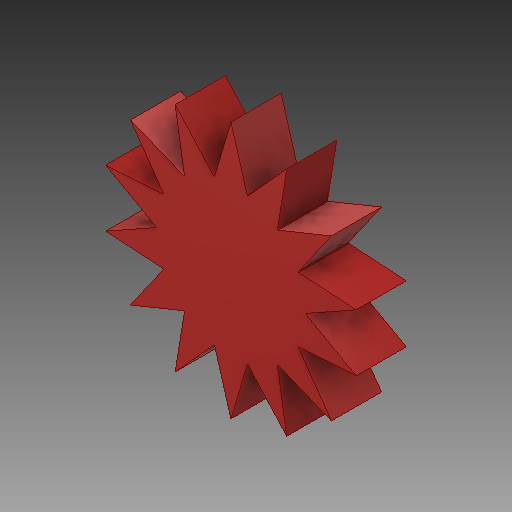
# Autodesk Inventor part: Small Gear Phone Case Mech
Saved by Autodesk Inventor 2018 (Build 220112000, 112)
## iProperties
Created: 2018-09-18
Part Number: Small Gear Phone Case Mech
Material: Generic
Document SubType Name: Modeling
Designer: User
Density: 1 g/cm^3
Appearance: Orange-Red
Author: User
Autodesk Inventor part; units mm, degrees
ref_plane "YZ Plane" through (0, 0, 0) normal (1, 0, 0) x (0, 1, 0)
ref_plane "XZ Plane" through (0, 0, 0) normal (0, 1, 0) x (-1, 0, 0)
ref_plane "XY Plane" through (0, 0, 0) normal (0, 0, 1) x (1, 0, 0)
sketch "Sketch1" plane through (0, 0, 0) normal (0, 0, 1) x (1, 0, 0)
  line L0 (-1.5495, 0.6331) -> (-0.724, 3.4271)
  line L1 (-0.724, 3.4271) -> (0.1015, 0.6331)
  line L2 (0.1015, 0.6331) -> (-1.5495, 0.6331) construction
  line L3 (-0.724, 0.6331) -> (-0.724, 0.8628) construction
  line L4 (-3.0816, -0.0934) -> (-3.5501, 2.7821)
  line L5 (-3.5501, 2.7821) -> (-1.5941, 0.623)
  line L6 (-4.1468, -1.4127) -> (-5.8165, 0.9748)
  line L7 (-5.8165, 0.9748) -> (-3.1174, -0.1219)
  line L8 (-4.534, -3.0635) -> (-7.0742, -1.637)
  line L9 (-7.0742, -1.637) -> (-4.1666, -1.4539)
  line L10 (-4.1666, -4.7188) -> (-7.0742, -4.5357)
  line L11 (-7.0742, -4.5357) -> (-4.534, -3.1092)
  line L12 (-3.1174, -6.0508) -> (-5.8165, -7.1474)
  line L13 (-5.8165, -7.1474) -> (-4.1468, -4.76)
  line L14 (-1.5941, -6.7957) -> (-3.5501, -8.9548)
  line L15 (-3.5501, -8.9548) -> (-3.0816, -6.0793)
  line L16 (0.1015, -6.8058) -> (-0.724, -9.5998)
  line L17 (-0.724, -9.5998) -> (-1.5495, -6.8058)
  line L18 (1.6335, -6.0793) -> (2.1021, -8.9548)
  line L19 (2.1021, -8.9548) -> (0.146, -6.7957)
  line L20 (2.6987, -4.76) -> (4.3684, -7.1474)
  line L21 (4.3684, -7.1474) -> (1.6693, -6.0508)
  line L22 (3.0859, -3.1092) -> (5.6261, -4.5357)
  line L23 (5.6261, -4.5357) -> (2.7185, -4.7188)
  line L24 (2.7185, -1.4539) -> (5.6261, -1.637)
  line L25 (5.6261, -1.637) -> (3.0859, -3.0635)
  line L26 (1.6693, -0.1219) -> (4.3684, 0.9748)
  line L27 (4.3684, 0.9748) -> (2.6987, -1.4127)
  line L28 (0.146, 0.623) -> (2.1021, 2.7821)
  line L29 (2.1021, 2.7821) -> (1.6335, -0.0934)
  arc A0 (-1.5495, 0.6331) -> (-1.5941, 0.623) centre (-0.724, -3.0863) ccw
  arc A1 (-3.0816, -0.0934) -> (-3.1174, -0.1219) centre (-0.724, -3.0863) ccw
  arc A2 (-4.1468, -1.4127) -> (-4.1666, -1.4539) centre (-0.724, -3.0863) ccw
  arc A3 (-4.534, -3.0635) -> (-4.534, -3.1092) centre (-0.724, -3.0863) ccw
  arc A4 (-4.1666, -4.7188) -> (-4.1468, -4.76) centre (-0.724, -3.0863) ccw
  arc A5 (-3.1174, -6.0508) -> (-3.0816, -6.0793) centre (-0.724, -3.0863) ccw
  arc A6 (-1.5941, -6.7957) -> (-1.5495, -6.8058) centre (-0.724, -3.0863) ccw
  arc A7 (0.1015, -6.8058) -> (0.146, -6.7957) centre (-0.724, -3.0863) ccw
  arc A8 (1.6335, -6.0793) -> (1.6693, -6.0508) centre (-0.724, -3.0863) ccw
  arc A9 (2.6987, -4.76) -> (2.7185, -4.7188) centre (-0.724, -3.0863) ccw
  arc A10 (3.0859, -3.1092) -> (3.0859, -3.0635) centre (-0.724, -3.0863) ccw
  arc A11 (2.7185, -1.4539) -> (2.6987, -1.4127) centre (-0.724, -3.0863) ccw
  arc A12 (1.6693, -0.1219) -> (1.6335, -0.0934) centre (-0.724, -3.0863) ccw
  arc A13 (0.146, 0.623) -> (0.1015, 0.6331) centre (-0.724, -3.0863) ccw
  point P0 (0, 0)
  dimension "d0" = 1.651
  dimension "d1" = 2.794
  constraints: 60 end point, 28 point on circle, 14 centre point, 1 horizontal, 1 midpoint, 1 vertical, 72 other
  measures "d0" distance of L0.start L1.end
  measures "d1" distance from line of L2 L0.end
extrude "Extrusion1" add sketch "Sketch1" along normal blind 2.54
body "Solid1"
